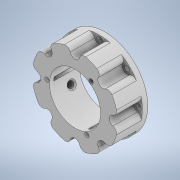
# Autodesk Inventor part: MotorHolder
Saved by Autodesk Inventor 2021 (Build 250183000, 183)
## iProperties
Created: 2021-02-09
Part Number: MotorHolder
Material: Generic
Document SubType Name: Modeling
Designer: Timo
Density: 1 g/cm^3
Appearance: Default
Author: Timo
Autodesk Inventor part; units mm, degrees
ref_plane "XZ Plane" through (0, 0, 0) normal (0, 1, 0) x (-1, 0, 0)
ref_plane "XY Plane" through (0, 0, 0) normal (0, 0, 1) x (1, 0, 0)
sketch "Sketch1" plane through (0, 0, 0) normal (0, 0, 1) x (1, 0, 0)
  circle A0 centre (0, 0) radius 35
  circle A1 centre (0, 0) radius 20.875
  dimension "d0" = 70
  dimension "d1" = 41.75
  constraints: 2 centre point, 2 coincident
  measures "d0" diameter of A0
  measures "d1" diameter of A1
extrude "Extrusion1" add sketch "Sketch1" along normal blind 24.45
sketch "Sketch2" plane through (0, 0, 24.45) normal (0, 0, 1) x (1, 0, 0)
  circle A0 centre (0, 0) radius 32 construction
  point P0 (0, 32)
  dimension "d4" = 64
  constraints: 1 coincident, 1 vertical alignment, 2 other
hole "Hole1" at (0, 32, 24.45) direction (0, 0, -1) diameter 4.5 end through all counterbore diameter 8 counterbore depth 20 clearance for "Socket Head Cap Screw" size "M4" standard "Ansi Metric M Profile"
fillet "Fillet1" radius 4 2 edges at (-2.7648, 34.8906, 14.45) (2.7648, 34.8906, 14.45)
pattern_circular "Circular Pattern1" count 8 over 360 about axis through (0, 0, -10) along (0, 0, 1) of "Hole1", "Fillet1"
ref_plane "Work Plane1" through (0, 0, 0) normal (0.9239, 0.3827, 0) x (0, 0, 1)
sketch "Sketch3" plane through (0, 0, 0) normal (0.9239, 0.3827, 0) x (0, 0, 1)
  circle A0 centre (8, 0) radius 2.5
  line L0 (0, -35) -> (0, 35) projected
  line L1 (-2.1, 0) -> (12.6, 0) projected
  point P0 (0, 0)
  dimension "d17" = 8
  dimension "d18" = 5
  constraints: 1 centre point, 1 point on line
  measures "d17" distance from line of A0.centre L0
  measures "d18" diameter of A0
extrude "Extrusion2" cut sketch "Sketch3" against normal through all
sketch "Sketch4" plane through (0, 0, 24.45) normal (0, 0, 1) x (1, 0, 0)
  circle A0 centre (0, 0) radius 23 construction
  circle A1 centre (13.1923, 18.8405) radius 1.75
  line L0 (0, -49) -> (0, 49) projected
  line L1 (13.1923, 18.8405) -> (0, 0) construction
  dimension "d21" = 46
  dimension "d22" = 3.5
  dimension "d31" = 35
  constraints: 2 end point, 1 centre point, 1 coincident, 3 other
  measures "d22" diameter of A1
  measures "d31" angle of L0 L1
extrude "Extrusion3" cut sketch "Sketch4" against normal blind 40.75
sketch "Sketch5" plane through (0, 0, 0) normal (0, 0, -1) x (-1, 0, 0)
  circle A0 centre (-13.1923, 18.8405) radius 1.75 projected
  line L0 (-11.6623, 16.1905) -> (-14.7222, 16.1905)
  line L1 (-14.7222, 16.1905) -> (-16.2522, 18.8405)
  line L2 (-16.2522, 18.8405) -> (-14.7222, 21.4905)
  line L3 (-14.7222, 21.4905) -> (-11.6623, 21.4905)
  line L4 (-11.6623, 21.4905) -> (-10.1323, 18.8405)
  line L5 (-10.1323, 18.8405) -> (-11.6623, 16.1905)
  point P0 (0, 0)
  dimension "d25" = 5.3
  constraints: 12 end point, 1 coincident, 1 horizontal, 13 other
  measures "d25" distance between parallel lines of L4 L1
extrude "Extrusion4" cut sketch "Sketch5" against normal blind 21
pattern_circular "Circular Pattern2" count 3 over 360 about axis through (0, 0, -10) along (0, 0, 1) of "Extrusion3", "Extrusion4"
chamfer "Chamfer1" distance 1 angle 45 1 edges at (-18.8893, -8.886, 5.7005)
sketch "Sketch6" plane through (-21.3825, -0.6454, 21) normal (0, 0, -1) x (-1, 0, 0)
  circle A0 centre (-21.3825, 0.6454) radius 21.25
  circle A1 centre (-31.1027, -20.1997) radius 1.75 projected
  circle A2 centre (-21.3825, 0.6454) radius 24.75
  circle A3 centre (1.53, 2.65) radius 1.75 projected
  circle A4 centre (-34.5748, 19.4859) radius 1.75 projected
  point P0 (-21.3825, 0.6454)
  constraints: 4 tangent, 2 centre point, 1 coincident
extrude "Extrusion5" add sketch "Sketch6" against normal blind 0.2 contours A0 A3 A2 A1 | A0 A4 A2 A3 | A3 | A1 A2 A4 A0 | A1 | A4
body "Solid1"
